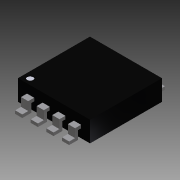
# Autodesk Inventor part: s74LVC2G08 Dual AND
Saved by Autodesk Inventor 2015 (Build 190159000, 159)
## iProperties
Created: 2016-01-19
Part Number: s74LVC2G08 Dual AND
Material: Generic
Document SubType Name: Modeling
Designer: Kyle
Density: 1 g/cm^3
Appearance: Default
Author: Kyle
Autodesk Inventor part; units mm, degrees
ref_plane "YZ Plane" through (0, 0, 0) normal (1, 0, 0) x (0, 1, 0)
ref_plane "XZ Plane" through (0, 0, 0) normal (0, 1, 0) x (-1, 0, 0)
ref_plane "XY Plane" through (0, 0, 0) normal (0, 0, 1) x (1, 0, 0)
sketch "Sketch1" plane through (0, 0, 0) normal (0, 0, 1) x (1, 0, 0)
  line L0 (0, 0) -> (2.9997, 0)
  line L1 (2.9997, 0) -> (2.9997, 0.8509)
  line L2 (2.9997, 0.8509) -> (0, 0.8509)
  line L3 (0, 0.8509) -> (0, 0)
  dimension "d0" = 2.9997
  dimension "d1" = 0.8509
  constraints: 8 end point, 2 parallel, 1 horizontal, 1 perpendicular
  measures "d0" distance of L1.end L2.end
  measures "d1" distance of L0.end L1.end
extrude "Extrusion1" add sketch "Sketch1" along normal blind 2.9972
sketch "Sketch2" plane through (0, 0, 2.9972) normal (0, 0, 1) x (1, 0, 0)
  line L0 (0.3759, 0.4839) -> (0.6756, 0.4839)
  line L1 (0.6756, 0.4839) -> (0.6756, 0.3543)
  line L2 (0.6756, 0.3543) -> (0.3759, 0.3543)
  line L3 (0.3759, 0.3543) -> (0.3759, 0.4839)
  line L4 (0, 0.8509) -> (0, 0) projected
  line L5 (2.9997, 0.8509) -> (0, 0.8509) projected
  line L6 (1.0262, 0.4839) -> (1.3259, 0.4839)
  line L7 (1.3259, 0.4839) -> (1.3259, 0.3543)
  line L8 (1.3259, 0.3543) -> (1.0262, 0.3543)
  line L9 (1.0262, 0.3543) -> (1.0262, 0.4839)
  line L10 (1.6764, 0.4839) -> (1.9761, 0.4839)
  line L11 (1.9761, 0.4839) -> (1.9761, 0.3543)
  line L12 (1.9761, 0.3543) -> (1.6764, 0.3543)
  line L13 (1.6764, 0.3543) -> (1.6764, 0.4839)
  line L14 (2.3266, 0.4839) -> (2.6264, 0.4839)
  line L15 (2.6264, 0.4839) -> (2.6264, 0.3543)
  line L16 (2.6264, 0.3543) -> (2.3266, 0.3543)
  line L17 (2.3266, 0.3543) -> (2.3266, 0.4839)
  dimension "d4" = 0.1295
  dimension "d5" = 0.2997
  dimension "d6" = 0.3759
  dimension "d7" = 0.367
  dimension "d10" = 0.6502
  constraints: 32 end point, 2 horizontal, 2 parallel, 1 perpendicular, 24 other
  measures "d4" distance of L0.end L1.end
  measures "d5" distance of L0.start L0.end
  measures "d6" distance between parallel lines of L3 L4
  measures "d7" distance between parallel lines of L5 L0
  measures "d10" distance of L0.start L6.start
extrude "Extrusion2" add sketch "Sketch2" along normal blind 0.1194
extrude "Extrusion3" add sketch "Sketch2" against normal blind 3.1166
sketch "Sketch3" plane through (0, 0, 3.1166) normal (0, 0, 1) x (1, 0, 0)
  line L0 (0.6756, 0.4839) -> (0.3759, 0.4839)
  line L1 (0.3759, 0.4839) -> (0.3759, 0.3543)
  line L2 (0.3759, 0.3543) -> (0.6756, 0.3543)
  line L3 (0.6756, 0.3543) -> (0.6756, 0.4839)
  line L4 (1.3259, 0.4839) -> (1.0262, 0.4839)
  line L5 (1.0262, 0.4839) -> (1.0262, 0.3543)
  line L6 (1.0262, 0.3543) -> (1.3259, 0.3543)
  line L7 (1.3259, 0.3543) -> (1.3259, 0.4839)
  line L8 (1.9761, 0.4839) -> (1.6764, 0.4839)
  line L9 (1.6764, 0.4839) -> (1.6764, 0.3543)
  line L10 (1.6764, 0.3543) -> (1.9761, 0.3543)
  line L11 (1.9761, 0.3543) -> (1.9761, 0.4839)
  line L12 (2.6264, 0.4839) -> (2.3266, 0.4839)
  line L13 (2.3266, 0.4839) -> (2.3266, 0.3543)
  line L14 (2.3266, 0.3543) -> (2.6264, 0.3543)
  line L15 (2.6264, 0.3543) -> (2.6264, 0.4839)
  point P0 (0, 0)
  constraints: 32 end point, 8 parallel, 4 horizontal, 4 perpendicular
extrude "Extrusion4" add sketch "Sketch3" along normal blind 0.1295
sketch "Sketch4" plane through (0, 0, -0.1194) normal (0, 0, -1) x (-1, 0, 0)
  line L0 (-2.6264, 0.4839) -> (-2.3266, 0.4839)
  line L1 (-2.3266, 0.4839) -> (-2.3266, 0.3543)
  line L2 (-2.3266, 0.3543) -> (-2.6264, 0.3543)
  line L3 (-2.6264, 0.3543) -> (-2.6264, 0.4839)
  line L4 (-1.9761, 0.4839) -> (-1.6764, 0.4839)
  line L5 (-1.6764, 0.4839) -> (-1.6764, 0.3543)
  line L6 (-1.6764, 0.3543) -> (-1.9761, 0.3543)
  line L7 (-1.9761, 0.3543) -> (-1.9761, 0.4839)
  line L8 (-1.3259, 0.4839) -> (-1.0262, 0.4839)
  line L9 (-1.0262, 0.4839) -> (-1.0262, 0.3543)
  line L10 (-1.0262, 0.3543) -> (-1.3259, 0.3543)
  line L11 (-1.3259, 0.3543) -> (-1.3259, 0.4839)
  line L12 (-0.6756, 0.4839) -> (-0.3759, 0.4839)
  line L13 (-0.3759, 0.4839) -> (-0.3759, 0.3543)
  line L14 (-0.3759, 0.3543) -> (-0.6756, 0.3543)
  line L15 (-0.6756, 0.3543) -> (-0.6756, 0.4839)
  point P0 (0, 0)
  constraints: 32 end point, 8 parallel, 4 horizontal, 4 perpendicular
extrude "Extrusion5" add sketch "Sketch4" along normal blind 0.1295
sketch "Sketch5" plane through (0.3759, 0.3543, 0) normal (0, -1, 0) x (1, 0, 0)
  line L0 (0.2997, 0) -> (0.2997, -0.2489) projected
  line L1 (0, -0.2489) -> (0.2997, -0.2489)
  line L2 (0.2997, -0.2489) -> (0.2997, -0.1245)
  line L3 (0.2997, -0.1245) -> (0, -0.1245)
  line L4 (0, -0.1245) -> (0, -0.2489)
  line L5 (0.95, 0) -> (0.95, -0.2489) projected
  line L6 (0.6502, -0.2489) -> (0.95, -0.2489)
  line L7 (0.95, -0.2489) -> (0.95, -0.1245)
  line L8 (0.95, -0.1245) -> (0.6502, -0.1245)
  line L9 (0.6502, -0.1245) -> (0.6502, -0.2489)
  line L10 (1.3005, -0.2489) -> (1.6002, -0.2489)
  line L11 (1.6002, -0.2489) -> (1.6002, -0.1245)
  line L12 (1.6002, -0.1245) -> (1.3005, -0.1245)
  line L13 (1.3005, -0.1245) -> (1.3005, -0.2489)
  line L14 (2.2504, 0) -> (2.2504, -0.2489) projected
  line L15 (1.9507, -0.2489) -> (2.2504, -0.2489)
  line L16 (2.2504, -0.2489) -> (2.2504, -0.1245)
  line L17 (2.2504, -0.1245) -> (1.9507, -0.1245)
  line L18 (1.9507, -0.1245) -> (1.9507, -0.2489)
  line L19 (0.2997, 2.9972) -> (0.2997, 3.2461) projected
  line L20 (0, 3.2461) -> (0.2997, 3.2461)
  line L21 (0.2997, 3.2461) -> (0.2997, 3.1217)
  line L22 (0.2997, 3.1217) -> (0, 3.1217)
  line L23 (0, 3.1217) -> (0, 3.2461)
  line L24 (0.95, 2.9972) -> (0.95, 3.2461) projected
  line L25 (0.6502, 3.2461) -> (0.95, 3.2461)
  line L26 (0.95, 3.2461) -> (0.95, 3.1217)
  line L27 (0.95, 3.1217) -> (0.6502, 3.1217)
  line L28 (0.6502, 3.1217) -> (0.6502, 3.2461)
  line L29 (1.6002, 2.9972) -> (1.6002, 3.2461) projected
  line L30 (1.3005, 3.2461) -> (1.6002, 3.2461)
  line L31 (1.6002, 3.2461) -> (1.6002, 3.1217)
  line L32 (1.6002, 3.1217) -> (1.3005, 3.1217)
  line L33 (1.3005, 3.1217) -> (1.3005, 3.2461)
  line L34 (2.2504, 2.9972) -> (2.2504, 3.2461) projected
  line L35 (1.9507, 3.2461) -> (2.2504, 3.2461)
  line L36 (2.2504, 3.2461) -> (2.2504, 3.1217)
  line L37 (2.2504, 3.1217) -> (1.9507, 3.1217)
  line L38 (1.9507, 3.1217) -> (1.9507, 3.2461)
  point P0 (-0.3759, 0)
  constraints: 64 end point, 16 parallel, 8 horizontal, 8 perpendicular, 7 midpoint, 1 point on line
extrude "Extrusion6" add sketch "Sketch5" along normal blind 0.3556
sketch "Sketch6" plane through (0, 0, 3.2461) normal (0, 0, 1) x (1, 0, 0)
  line L0 (0.3759, 0.4839) -> (0.3759, -0.0013) projected
  line L1 (0.6756, -0.0013) -> (0.3759, -0.0013)
  line L2 (0.3759, -0.0013) -> (0.3759, 0.1283)
  line L3 (0.3759, 0.1283) -> (0.6756, 0.1283)
  line L4 (0.6756, 0.1283) -> (0.6756, -0.0013)
  line L5 (1.3259, 0.3543) -> (1.3259, -0.0013) projected
  line L6 (1.0262, -0.0013) -> (1.3259, -0.0013)
  line L7 (1.3259, -0.0013) -> (1.3259, 0.1283)
  line L8 (1.3259, 0.1283) -> (1.0262, 0.1283)
  line L9 (1.0262, 0.1283) -> (1.0262, -0.0013)
  line L10 (1.9761, 0.3543) -> (1.9761, -0.0013) projected
  line L11 (1.6764, -0.0013) -> (1.9761, -0.0013)
  line L12 (1.9761, -0.0013) -> (1.9761, 0.1283)
  line L13 (1.9761, 0.1283) -> (1.6764, 0.1283)
  line L14 (1.6764, 0.1283) -> (1.6764, -0.0013)
  line L15 (2.6264, 0.4839) -> (2.6264, -0.0013) projected
  line L16 (2.3266, -0.0013) -> (2.6264, -0.0013)
  line L17 (2.6264, -0.0013) -> (2.6264, 0.1283)
  line L18 (2.6264, 0.1283) -> (2.3266, 0.1283)
  line L19 (2.3266, 0.1283) -> (2.3266, -0.0013)
  point P0 (0, 0)
  dimension "d25" = 0.1295
  constraints: 32 end point, 8 parallel, 6 point on line, 4 horizontal, 4 perpendicular
  measures "d25" distance between parallel lines of L1 L3
extrude "Extrusion7" add sketch "Sketch6" along normal blind 0.2464
sketch "Sketch7" plane through (0, 0, -0.2489) normal (0, 0, -1) x (-1, 0, 0)
  line L0 (-2.6264, -0.0013) -> (-2.3266, -0.0013)
  line L1 (-2.3266, -0.0013) -> (-2.3266, 0.1283)
  line L2 (-2.3266, 0.1283) -> (-2.6264, 0.1283)
  line L3 (-2.6264, 0.1283) -> (-2.6264, -0.0013)
  line L4 (-1.9761, -0.0013) -> (-1.6764, -0.0013)
  line L5 (-1.6764, -0.0013) -> (-1.6764, 0.1283)
  line L6 (-1.6764, 0.1283) -> (-1.9761, 0.1283)
  line L7 (-1.9761, 0.1283) -> (-1.9761, -0.0013)
  line L8 (-1.0262, 0.3543) -> (-1.0262, -0.0013) projected
  line L9 (-1.3259, -0.0013) -> (-1.0262, -0.0013)
  line L10 (-1.0262, -0.0013) -> (-1.0262, 0.1283)
  line L11 (-1.0262, 0.1283) -> (-1.3259, 0.1283)
  line L12 (-1.3259, 0.1283) -> (-1.3259, -0.0013)
  line L13 (-0.6756, -0.0013) -> (-0.3759, -0.0013)
  line L14 (-0.3759, -0.0013) -> (-0.3759, 0.1283)
  line L15 (-0.3759, 0.1283) -> (-0.6756, 0.1283)
  line L16 (-0.6756, 0.1283) -> (-0.6756, -0.0013)
  point P0 (0, 0)
  constraints: 32 end point, 8 parallel, 4 horizontal, 4 perpendicular, 2 point on line
extrude "Extrusion8" add sketch "Sketch7" along normal blind 0.2464
sketch "Sketch8" plane through (0, 0, 0) normal (0, -1, 0) x (1, 0, 0)
  line L0 (-1.2528, -0.9199) -> (4.4304, -0.9199)
  line L1 (4.4304, -0.9199) -> (4.4304, 4.3493)
  line L2 (4.4304, 4.3493) -> (-1.2528, 4.3493)
  line L3 (-1.2528, 4.3493) -> (-1.2528, -0.9199)
  point P0 (0, 0)
  constraints: 8 end point, 2 parallel, 1 horizontal, 1 perpendicular
extrude "Extrusion9" cut sketch "Sketch8" along normal blind 0.2464
sketch "Sketch9" plane through (0, 0.8509, 0) normal (0, 1, 0) x (1, 0, 0)
  circle A0 centre (0.254, -2.7432) radius 0.127
  line L0 (2.9997, -2.9972) -> (0, -2.9972) projected
  line L1 (0, 0) -> (0, -2.9972) projected
  dimension "d32" = 0.254
  dimension "d33" = 0.254
  dimension "d34" = 0.254
  constraints: 1 centre point
  measures "d32" diameter of A0
  measures "d33" distance from line of L0 A0.centre
  measures "d34" distance from line of L1 A0.centre
extrude "Extrusion10" cut sketch "Sketch9" against normal blind 0.0254
body "Solid1"
